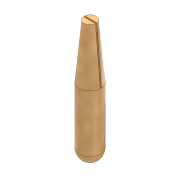
# Autodesk Inventor part: PMECAD_LEGOmini_FlagFrame
Saved by Autodesk Inventor 2018.3 (Build 223284000, 284)
## iProperties
Created: 2019-02-01
Part Number: PMECAD_LEGOmini_FlagFrame
Material: 松木、赤松
Document SubType Name: Modeling
Designer: 賢賢
Density: 0.496 g/cm^3
Appearance: 黃色松木 - 深色中亮度
Author: 賢賢
Autodesk Inventor part; units mm, degrees
ref_plane "YZ Plane" through (0, 0, 0) normal (1, 0, 0) x (0, 1, 0)
ref_plane "XZ Plane" through (0, 0, 0) normal (0, 1, 0) x (-1, 0, 0)
ref_plane "XY Plane" through (0, 0, 0) normal (0, 0, 1) x (1, 0, 0)
sketch "草圖1" plane through (0, 0, 0) normal (0, 0, 1) x (1, 0, 0)
  circle A0 centre (0, 0) radius 1.6
  dimension "d0" = 3.2
  constraints: 1 centre point, 1 coincident
  measures "d0" diameter of A0
extrude "擠出1" add sketch "草圖1" along normal blind 10
sketch "草圖2" plane through (0, 0, 10) normal (0, 0, 1) x (1, 0, 0)
  line L0 (2.5, -0.1) -> (-2.5, -0.1)
  line L1 (-2.5, -0.1) -> (-2.5, 0.1)
  line L2 (-2.5, 0.1) -> (2.5, 0.1)
  line L3 (2.5, 0.1) -> (2.5, -0.1)
  line L4 (2.5, -0.1) -> (-2.5, 0.1) construction
  line L5 (-2.5, -0.1) -> (2.5, 0.1) construction
  point P0 (0, 0)
  dimension "d3" = 5
  dimension "d4" = 0.2
  constraints: 12 end point, 2 midpoint, 2 parallel, 1 horizontal, 1 perpendicular
  measures "d3" distance of L1.end L2.end
  measures "d4" distance of L0.end L1.end
sketch "草圖3" plane through (0, 0, 10) normal (0, 0, 1) x (1, 0, 0)
  circle A0 centre (0, 0) radius 1.6 projected
extrude "擠出2" add sketch "草圖3" along normal blind 8 draft -5
extrude "擠出3" cut sketch "草圖2" along normal through all
fillet "圓角1" radius 1.6 1 edges at (-1.6, 0, 0)
